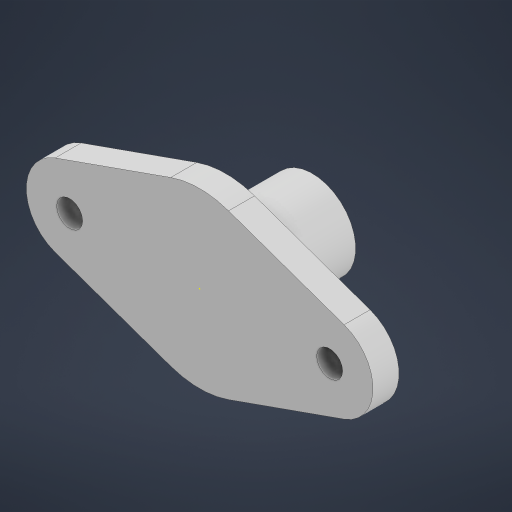
# Autodesk Inventor part: ServoDrive
Saved by Autodesk Inventor 2023 (Build 270158000, 158)
## iProperties
Created: 2023-02-24
Part Number: ServoDrive
Material: Generic
Document SubType Name: Modeling
Designer: roota
Density: 1 g/cm^3
Appearance: Default
Author: roota
Autodesk Inventor part; units mm, degrees
ref_plane "YZ Plane" through (0, 0, 0) normal (1, 0, 0) x (0, 1, 0)
ref_plane "XZ Plane" through (0, 0, 0) normal (0, 1, 0) x (-1, 0, 0)
ref_plane "XY Plane" through (0, 0, 0) normal (0, 0, 1) x (1, 0, 0)
sketch "Sketch1" plane through (0, 0, 0) normal (0, 0, 1) x (1, 0, 0)
  circle A0 centre (0, 0) radius 10
  circle A1 centre (15, 0) radius 5
  circle A2 centre (-15, 0) radius 5
  line L0 (-16.6667, 4.714) -> (-3.3333, 9.4281)
  line L1 (-16.6667, -4.714) -> (-3.3333, -9.4281)
  line L2 (3.3333, -9.4281) -> (16.6667, -4.714)
  line L3 (16.6667, 4.714) -> (3.3333, 9.4281)
  dimension "d0" = 20
  dimension "d1" = 10
  dimension "d2" = 10
  dimension "d3" = 15
  dimension "d4" = 15
  constraints: 8 end point, 8 point on circle, 8 tangent, 3 centre point, 2 horizontal alignment, 1 coincident
  measures "d0" diameter of A0
  measures "d1" diameter of A1
  measures "d2" diameter of A2
  measures "d3" distance of point (0, 0) A1.centre
  measures "d4" distance of point (0, 0) A2.centre
extrude "Extrusion1" add sketch "Sketch1" along normal blind 3
sketch "Sketch2" plane through (0, 0, 0) normal (0, 0, -1) x (-1, 0, 0)
  circle A0 centre (0, 0) radius 5
  dimension "d7" = 10
  constraints: 1 centre point, 1 coincident
  measures "d7" diameter of A0
extrude "Extrusion2" add sketch "Sketch2" along normal blind 10
sketch "Sketch3" plane through (0, 0, 3) normal (0, 0, 1) x (1, 0, 0)
  point P0 (0, 0)
sketch "Sketch4" plane through (0, 0, 3) normal (0, 0, 1) x (1, 0, 0)
  arc A0 (-16.6667, 4.714) -> (-16.6667, -4.714) centre (-15, 0) ccw projected
  circle A1 centre (-15, 0) radius 1.5
  arc A2 (16.6667, -4.714) -> (16.6667, 4.714) centre (15, 0) ccw projected
  circle A3 centre (15, 0) radius 1.5
  point P0 (0, 0)
  dimension "d10" = 3
  dimension "d11" = 3
  constraints: 2 centre point, 2 coincident
  measures "d10" diameter of A1
  measures "d11" diameter of A3
extrude "Extrusion3" cut sketch "Sketch4" against normal through all
equation "\"d4\" = d3"
body "Solid1"
